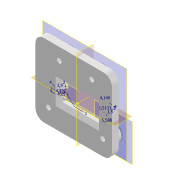
# Autodesk Inventor part: Cover_new
Saved by Autodesk Inventor 2022 (Build 260153000, 153)
## iProperties
Created: 2021-06-04
Part Number: Cover_new
Material: Generic
Document SubType Name: Modeling
Designer: wanghaoran
Density: 1 g/cm^3
Appearance: Default
Author: wanghaoran
Autodesk Inventor part; units mm, degrees
ref_plane "YZ Plane" through (0, 0, 0) normal (1, 0, 0) x (0, 1, 0)
ref_plane "XZ Plane" through (0, 0, 0) normal (0, 1, 0) x (-1, 0, 0)
ref_plane "XY Plane" through (0, 0, 0) normal (0, 0, 1) x (1, 0, 0)
sketch "Sketch1" plane through (0, 0, 0) normal (0, 0, 1) x (1, 0, 0)
  line L0 (0, 0) -> (45, 0)
  line L1 (45, 0) -> (45, 43)
  line L2 (45, 43) -> (0, 43)
  line L3 (0, 43) -> (0, 0)
  line L4 (13.851, 13.85) -> (35.351, 13.85)
  line L5 (35.351, 13.85) -> (35.351, 25.05)
  line L6 (35.351, 25.05) -> (13.851, 25.05)
  line L7 (13.851, 25.05) -> (13.851, 13.85)
  dimension "d0" = 45
  dimension "d1" = 43
  dimension "d2" = 21.5
  dimension "d3" = 11.2
  dimension "d4" = 9.649
  dimension "d16" = 17.95
  constraints: 16 end point, 4 parallel, 2 horizontal, 2 perpendicular
  measures "d0" distance of L2.end L1.end
  measures "d1" distance of L1.end L0.end
  measures "d2" distance of L6.end L5.end
  measures "d3" distance of L5.end L4.end
  measures "d4" distance between parallel lines of L1 L5
  measures "d16" distance between parallel lines of L2 L6
extrude "Extrusion1" add sketch "Sketch1" along normal blind 4
fillet "Fillet1" radius 5 4 edges at (45, 43, 2) (45, 0, 2) (0, 43, 2) (0, 0, 2)
ref_plane "Work Plane1" through (0, 0, -2.5) normal (0, 0, -1) x (-1, 0, 0)
sketch "Sketch2" plane through (0, 0, 4) normal (0, 0, 1) x (1, 0, 0)
  circle A0 centre (14.02, 35.95) radius 1.4
  circle A1 centre (33.02, 35.95) radius 1.4
  line L0 (0, 43) -> (0, 0) projected
  line L1 (45, 0) -> (45, 43) projected
  line L2 (45, 43) -> (0, 43) projected
  circle A2 centre (7.52, 8.95) radius 1.4
  circle A3 centre (39.52, 8.95) radius 1.4
  line L3 (13.851, 13.85) -> (13.851, 25.05) projected
  line L4 (35.351, 13.85) -> (13.851, 13.85) projected
  line L5 (13.851, 25.05) -> (35.351, 25.05) projected
  dimension "d8" = 2.8
  dimension "d9" = 2.8
  dimension "d14" = 2.8
  dimension "d15" = 2.8
  dimension "d18" = 32
  dimension "d19" = 6.331
  dimension "d20" = 4.9
  dimension "d22" = 19
  dimension "d23" = 10.9
  dimension "d24" = 10.9
  dimension "d25" = 0.169
  dimension "d28" = 4.9
  constraints: 4 centre point
  measures "d8" diameter of A0
  measures "d9" diameter of A1
  measures "d14" diameter of A2
  measures "d15" diameter of A3
  measures "d18" distance of A3.centre A2.centre
  measures "d19" distance from line of L3 A2.centre
  measures "d20" distance from line of A2.centre L4
  measures "d22" distance of A1.centre A0.centre
  measures "d23" distance from line of L5 A0.centre
  measures "d24" distance from line of L5 A1.centre
  measures "d25" distance from line of L3 A0.centre
  measures "d28" distance from line of L4 A3.centre
extrude "Extrusion2" cut sketch "Sketch2" against normal through all
sketch "Sketch3" plane through (0, 0, 0) normal (0, 0, -1) x (-1, 0, 0)
  circle A0 centre (-39.52, 8.95) radius 1.4 projected
  circle A1 centre (-39.52, 8.95) radius 4.65
  circle A2 centre (-33.02, 35.95) radius 1.4 projected
  circle A3 centre (-33.02, 35.95) radius 4.65
  circle A4 centre (-14.02, 35.95) radius 1.4 projected
  circle A5 centre (-14.02, 35.95) radius 4.65
  circle A6 centre (-7.52, 8.95) radius 1.4 projected
  circle A7 centre (-7.52, 8.95) radius 4.65
  circle A8 centre (-39.52, 8.95) radius 1.4
  circle A9 centre (-7.52, 8.95) radius 1.4
  circle A10 centre (-14.02, 35.95) radius 1.4
  circle A11 centre (-33.02, 35.95) radius 1.4
  point P0 (0, 0)
  dimension "d30" = 9.3
  dimension "d31" = 9.3
  dimension "d32" = 9.3
  dimension "d33" = 9.3
  constraints: 8 centre point, 8 coincident, 4 concentric
  measures "d30" diameter of A1
  measures "d31" diameter of A3
  measures "d32" diameter of A5
  measures "d33" diameter of A7
sketch "Sketch4" plane through (0, 0, -2.5) normal (0, 0, -1) x (-1, 0, 0)
  circle A0 centre (-39.52, 8.95) radius 1.4 projected
  circle A1 centre (-7.52, 8.95) radius 1.4 projected
  circle A2 centre (-14.02, 35.95) radius 1.4 projected
  circle A3 centre (-33.02, 35.95) radius 1.4 projected
  circle A4 centre (-33.02, 35.95) radius 2.1
  circle A5 centre (-14.02, 35.95) radius 2.1
  circle A6 centre (-7.52, 8.95) radius 2.1
  circle A7 centre (-39.52, 8.95) radius 2.1
  point P0 (0, 0)
  dimension "d35" = 4.2
  dimension "d36" = 4.2
  dimension "d37" = 4.2
  dimension "d38" = 4.2
  constraints: 4 centre point, 4 coincident
  measures "d35" diameter of A4
  measures "d36" diameter of A5
  measures "d37" diameter of A6
  measures "d38" diameter of A7
ref_plane "Work Plane2" through (39.52, 8.95, -2.5) normal (0, 0, -1) x (-1, 0, 0)
ref_plane "Work Plane3" through (7.52, 8.95, -2.5) normal (0, 0, -1) x (-1, 0, 0)
sketch "Sketch6" plane through (7.52, 8.95, -2.5) normal (0, 0, -1) x (-1, 0, 0)
  circle A0 centre (0, 0) radius 1.4 projected
  circle A1 centre (0, 0) radius 2.15 projected
  circle A2 centre (-32, 0) radius 1.4 projected
  circle A3 centre (-32, 0) radius 2.15 projected
  circle A4 centre (-25.5, 27) radius 1.4 projected
  circle A5 centre (-25.5, 27) radius 2.15 projected
  circle A6 centre (-6.5, 27) radius 2.15 projected
  circle A7 centre (-6.5, 27) radius 1.4 projected
  point P0 (7.52, -8.95)
chamfer "Chamfer1" distance 2 angle 45 4 edges at (24.601, 13.85, 4) (35.351, 19.45, 4) (24.601, 25.05, 4) (13.851, 19.45, 4)
sketch "Sketch7" plane through (0, 0, 0) normal (0, 0, -1) x (-1, 0, 0)
  line L0 (-13.851, 13.85) -> (-35.351, 13.85) projected
  line L1 (-13.851, 25.05) -> (-13.851, 13.85) projected
  line L2 (-35.351, 25.05) -> (-13.851, 25.05) projected
  line L3 (-35.351, 13.85) -> (-35.351, 25.05) projected
  line L4 (-12.851, 18) -> (-11.851, 18)
  line L5 (-11.851, 18) -> (-11.851, 20.9)
  line L6 (-11.851, 20.9) -> (-12.851, 20.9)
  line L7 (-13.851, 19.9) -> (-13.851, 19)
  arc A0 (-13.851, 19) -> (-12.851, 18) centre (-12.851, 19) ccw
  arc A1 (-12.851, 20.9) -> (-13.851, 19.9) centre (-12.851, 19.9) ccw
  circle A2 centre (-36.864, 19.438) radius 0.75
  circle A3 centre (-39.5, 23.05) radius 0.65
  circle A4 centre (-9.3, 15.85) radius 0.65
  circle A5 centre (-9.3, 15.85) radius 2
  circle A6 centre (-39.5, 23.05) radius 2
  point P0 (0, 0)
  point P1 (-13.851, 18)
  point P2 (-13.851, 20.9)
  dimension "d70" = 2
  dimension "d71" = 2.9
  dimension "d72" = 4.15
  dimension "d73" = 1
  dimension "d74" = 1.5
  dimension "d75" = 1.513
  dimension "d76" = 5.588
  dimension "d77" = 4.149
  dimension "d78" = 1.3
  dimension "d79" = 2
  dimension "d80" = 1.3
  dimension "d81" = 4.551
  dimension "d82" = 2
  dimension "d87" = 4
  dimension "d88" = 4
  constraints: 8 end point, 7 centre point, 5 point on line, 4 point on circle, 4 tangent, 2 coincident, 2 parallel, 1 equal radius, 1 horizontal, 1 perpendicular
  measures "d70" distance of point (-13.851, 20.9) L5.end
  measures "d71" distance of L5.end L4.end
  measures "d72" distance between parallel lines of L0 L4
  measures "d73" radius of A0
  measures "d74" diameter of A2
  measures "d75" distance from line of L3 A2.centre
  measures "d76" distance from line of L0 A2.centre
  measures "d77" distance from line of L3 A3.centre
  measures "d78" diameter of A3
  measures "d79" distance from line of L2 A3.centre
  measures "d80" diameter of A4
  measures "d81" distance from line of L1 A4.centre
  measures "d82" distance from line of A4.centre L0
  measures "d87" diameter of A5
  measures "d88" diameter of A6
extrude "Extrusion5" add sketch "Sketch7" along normal blind 1.6 contours L1 A1 L6 L5 L4 A0 | A2 | A5 | A6
extrude "Extrusion6" add sketch "Sketch7" along normal blind 2.9 contours A3 | A4
extrude "Extrusion7" add sketch "Sketch3" along normal blind 3
extrude "Extrusion9" add sketch "Sketch4" along normal blind 2.6
ref_plane "Work Plane4" through (11.851, 19.45, -3.6) normal (0, 1, 0) x (-1, 0, 0)
ref_plane "Work Plane5" through (24.601, 11.85, -8.75) normal (1, 0, 0) x (0, 1, 0)
body "Solid1"
